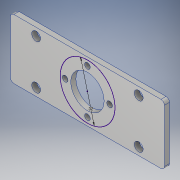
# Autodesk Inventor part: 板 中心Φ7
Saved by Autodesk Inventor 2019 (Build 230136000, 136)
## iProperties
Created: 2020-10-08
Part Number: 板 中心Φ7
Material: アルミニウム 6061
Document SubType Name: Modeling
Designer: zhept
Density: 2.7 g/cm^3
Appearance: アルミニウム - フラット
Author: zhept
Autodesk Inventor part; units mm, degrees
ref_plane "YZ Plane" through (0, 0, 0) normal (1, 0, 0) x (0, 1, 0)
ref_plane "XZ Plane" through (0, 0, 0) normal (0, 1, 0) x (-1, 0, 0)
ref_plane "XY Plane" through (0, 0, 0) normal (0, 0, 1) x (1, 0, 0)
sketch "スケッチ6" plane through (0, 0, 0) normal (0, 0, 1) x (1, 0, 0)
  line L0 (45, -17.5) -> (-45, -17.5)
  line L1 (-45, -17.5) -> (-45, 17.5)
  line L2 (-45, 17.5) -> (45, 17.5)
  line L3 (45, 17.5) -> (45, -17.5)
  line L4 (45, -17.5) -> (-45, 17.5) construction
  line L5 (-45, -17.5) -> (45, 17.5) construction
  point P0 (0, 0)
  dimension "d29" = 90
  dimension "d30" = 35
  constraints: 12 end point, 2 midpoint, 2 parallel, 1 horizontal, 1 perpendicular
  measures "d29" distance of L0.start L0.end
  measures "d30" distance of L0.end L1.end
extrude "押し出し6" add sketch "スケッチ6" along normal blind 3
sketch "スケッチ7" plane through (0, 0, 3) normal (0, 0, 1) x (1, 0, 0)
  circle A0 centre (0, 0) radius 9.75
  dimension "d33" = 19.5
  constraints: 1 centre point, 1 coincident
  measures "d33" diameter of A0
extrude "押し出し7" cut sketch "スケッチ7" against normal blind 3
sketch "スケッチ8" plane through (0, 0, 3) normal (0, 0, 1) x (1, 0, 0)
  circle A0 centre (0, 13) radius 1.65
  circle A1 centre (0, -13) radius 1.65
  circle A2 centre (13, 0) radius 1.65
  circle A3 centre (-13, 0) radius 1.65
  point P0 (0, 0)
  dimension "d36" = 3.3
  dimension "d37" = 3.3
  dimension "d38" = 3.3
  dimension "d39" = 3.3
  constraints: 4 centre point
  measures "d36" diameter of A0
  measures "d37" diameter of A1
  measures "d38" diameter of A2
  measures "d39" diameter of A3
extrude "押し出し8" cut sketch "スケッチ8" against normal blind 3
sketch "スケッチ9" plane through (0, 0, 3) normal (0, 0, 1) x (1, 0, 0)
  circle A0 centre (-30, 13) radius 2.6
  circle A1 centre (30, 13) radius 2.6
  circle A2 centre (-30, -13) radius 2.6
  circle A3 centre (30, -13) radius 2.6
  point P0 (0, 0)
  dimension "d50" = 5.2
  dimension "d51" = 5.2
  dimension "d52" = 5.2
  dimension "d53" = 5.2
  constraints: 4 centre point
  measures "d50" diameter of A0
  measures "d51" diameter of A1
  measures "d52" diameter of A2
  measures "d53" diameter of A3
sketch "スケッチ10" plane through (0, 0, 3) normal (0, 0, 1) x (1, 0, 0)
  circle A0 centre (0, 0) radius 16
  dimension "d43" = 32
  constraints: 1 centre point, 1 coincident
  measures "d43" diameter of A0
extrude "押し出し9" cut sketch "スケッチ9" against normal blind 3
fillet "フィレット1" radius 2 4 edges at (-45, 17.5, 1.5) (45, 17.5, 1.5) (45, -17.5, 1.5) (-45, -17.5, 1.5)
